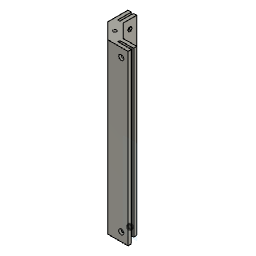
Pied_LEDcube (Autodesk Fusion 360 design; units mm, degrees)
Autodesk Fusion 360 part; units mm, degrees
sketch "Esquisse1" plane through (0, 0, 0) normal (0, 0, 1) x (1, 0, 0)
  line L0 (0, 0) -> (30, 0)
  line L1 (30, 0) -> (30, 5)
  line L2 (30, 5) -> (10, 5)
  line L3 (10, 5) -> (10, 8)
  line L4 (10, 8) -> (30, 8)
  line L5 (30, 8) -> (30, 13)
  line L6 (30, 13) -> (10, 13)
  line L7 (10, 13) -> (0, 23)
  line L8 (0, 23) -> (-11.5, 11.5)
  line L9 (-11.5, 11.5) -> (0, 0)
  dimension "d2" = 3
  dimension "d3" = 5
  dimension "d4" = 20
  dimension "d5" = 30
  dimension "d6" = 20
  dimension "d7" = 15
  dimension "d8" = 135
  dimension "d22" = 13
  constraint coincident L0.start L9.end
  constraint horizontal L0
  constraint perpendicular L0 L1
  constraint perpendicular L1 L2
  constraint perpendicular L2 L3
  constraint perpendicular L3 L4
  constraint perpendicular L2 L5
  constraint perpendicular L5 L6
  constraint perpendicular L7 L8
  constraint parallel L7 L9
  constraint equal L1 L5
  constraint equal L2 L4
  measures "d2" distance of L2.end L3.end
  measures "d3" distance of L0.end L1.end
  measures "d4" distance of L5.end L6.end
  measures "d5" distance of L0.start L0.end
  measures "d6" distance of L1.end L2.end
  measures "d7" distance of L4 L7.end
  measures "d8" angle of L6 L7
  measures "d22" distance of L0 L6
extrude "Extrusion1" add sketch "Esquisse1" along normal blind 125 makes body 1
chamfer "Chanfrein2" distance 2 angle 25 1 edges at (30, 8, 62.5) measured on face at (16.6667, 8, 41.6667) on bodies 1
sketch "Esquisse2" plane through (0, 0, 0) normal (0, -1, 0) x (1, 0, 0)
  line L0 (0, 0) -> (30, 0)
  line L1 (30, 0) -> (30, 125)
  line L2 (30, 125) -> (0, 125)
  line L3 (0, 125) -> (0, 0)
  circle A0 centre (20, 12.85) radius 1.7
  line L4 (18.3546, 15.7) -> (16.7091, 12.85)
  line L5 (16.7091, 12.85) -> (18.3546, 10)
  line L6 (18.3546, 10) -> (21.6454, 10)
  line L7 (21.6454, 10) -> (23.2909, 12.85)
  line L8 (23.2909, 12.85) -> (21.6454, 15.7)
  line L9 (21.6454, 15.7) -> (18.3546, 15.7)
  line L10 (0, 0) -> (30, 0)
  point P0 (20, 12.85)
  point P1 (-10, 0)
  point P2 (-30, 125)
  dimension "d11" = 3.4
  dimension "d12" = 2.85
  dimension "d15" = 10
  dimension "d16" = 10
  constraint coincident P0 A0.centre
  constraint parallel L6 L10
  measures "d11" diameter of A0
  measures "d12" distance of P0 L9
  measures "d15" distance of L1 P0
  measures "d16" distance of L6 L10
extrude "Extrusion2" cut sketch "Esquisse2" against normal blind 13 contours A0 bodies 1
chamfer "Chanfrein1" distance 2 angle 45 1 edges at (18.415, 0, 13.4647) on bodies 1
sketch "Esquisse3" plane through (0, 13, 0) normal (0, 1, 0) x (-1, 0, 0)
  circle A0 centre (-20, 12.85) radius 1.7
  line L0 (-30, 0) -> (-10, 0)
  line L1 (-10, 0) -> (-10, 125)
  line L2 (-10, 125) -> (-30, 125)
  line L3 (-30, 125) -> (-30, 0)
  line L4 (-18.3546, 15.7) -> (-21.6454, 15.7)
  line L5 (-21.6454, 15.7) -> (-23.2909, 12.85)
  line L6 (-23.2909, 12.85) -> (-21.6454, 10)
  line L7 (-21.6454, 10) -> (-18.3546, 10)
  line L8 (-18.3546, 10) -> (-16.7091, 12.85)
  line L9 (-16.7091, 12.85) -> (-18.3546, 15.7)
  point P0 (-20, 12.85)
  dimension "d23" = 2.85
  constraint coincident P0 A0.centre
  constraint parallel L0 L7
  measures "d23" distance of P0 L9
extrude "Extrusion4" cut sketch "Esquisse3" against normal blind 3 contours L4 L5 L6 L7 L8 L9 bodies 1
ref_plane "Plan de construction2" through (-5.75, 17.25, 62.5) normal (-0.707107, 0.707107, 0) x (-0.707107, -0.707107, 0)
mirror "Symétrie miroir1" about plane through (-5.75, 17.25, 62.5) normal (-0.707107, 0.707107, 0) of bodies 1 merged
sketch "Esquisse4" plane through (0, 0, 0) normal (0, 0, 1) x (1, 0, 0)
  line L0 (10, 13) -> (-10, 33) construction
  line L1 (-6.2132, 8) -> (-6.2132, 16.7868) construction
  line L2 (-6.2132, 16.7868) -> (-15, 16.7868) construction
  line L3 (-6.2132, 16.7868) -> (0, 23) construction
  line L4 (29.8, 8) -> (8.2, 8) construction
  line L5 (-15, 52.8) -> (-15, 31.2) construction
  circle A0 centre (-6.2132, 16.7868) radius 2.5
  point P0 (-15, 8)
  dimension "d32" = 5
  dimension "d33" = 8.7868
  constraint vertical L1
  constraint perpendicular L1 L2
  constraint equal L1 L2
  constraint coincident L0 L3.end
  constraint coincident L1.start L4
  constraint coincident L2.end L5
  constraint perpendicular L0 L3
  constraint equal L2 L3
  constraint coincident L1.end L2.start
  measures "d32" diameter of A0
  measures "d33" distance of L0 L1.end
extrude "Extrusion5" cut sketch "Esquisse4" along normal blind 35 bodies 1
ref_plane "Plan de construction3" through (3.5, 26.5, 125) normal (0, 0, 1) x (1, 0, 0)
mirror "Symétrie miroir2" about plane through (3.5, 26.5, 125) normal (0, 0, 1) of bodies 1 merged
sketch "Esquisse5" plane through (0, 0, 0) normal (0, 0, -1) x (1, 0, 0)
  line L0 (30, -8.9326) -> (28, -8)
  line L1 (28, -8) -> (10, -8)
  line L2 (10, -8) -> (10, -5)
  line L3 (10, -5) -> (30, -5)
  line L4 (30, -5) -> (30, 0)
  line L5 (30, 0) -> (0, 0)
  line L6 (0, 0) -> (-23, -23)
  line L7 (-23, -23) -> (-23, -53)
  line L8 (-23, -53) -> (-18, -53)
  line L9 (-18, -53) -> (-18, -33)
  line L10 (-18, -33) -> (-15, -33)
  line L11 (-15, -33) -> (-15, -51)
  line L12 (-15, -51) -> (-14.0674, -53)
  line L13 (-14.0674, -53) -> (-10, -53)
  line L14 (-10, -53) -> (-10, -33)
  line L15 (-10, -33) -> (10, -13)
  line L16 (10, -13) -> (30, -13)
  line L17 (30, -13) -> (30, -8.9326)
  line L18 (-15, -8) -> (185, -8)
  line L19 (185, -8) -> (185, -208)
  line L20 (185, -208) -> (-15, -208)
  line L21 (-15, -208) -> (-15, -8)
  circle A0 centre (-6.2132, -16.7868) radius 2.5
  dimension "d39" = 200
  dimension "d40" = 200
  constraint horizontal L18
  constraint vertical L19
  constraint horizontal L20
  constraint vertical L21
  measures "d39" distance of L18.start L18.end
  measures "d40" distance of L18.start L20.end
extrude "Extrusion6" cut sketch "Esquisse5" against normal blind 7 contours L0 L1 L6 L11 L12 L13 L14 L15 L16 L17 L18 L21 | L0 L12 L13 L14 L15 L16 L17 L18 L19 L20 L21 | A0 bodies 1
copy_body "Corps->Comp1" bodies 1 removing the originals makes body 2 in component "Component"
component "Component" placed x (1, 0, 0) y (0, 1, 0) z (0, 0, 1) at (0, 0, 0)
equation "d4 = d6 + 0 mm"
equation "d5 = d4 + 10 mm"
equation "d9 = ( 250 / 2 ) * 1 mm"
equation "d13 = -( 2 * d3 + d2 )"
equation "d15 = d6 / 2"
equation "d23 = d12"
equation "d27 = -d3 + 2 mm"
